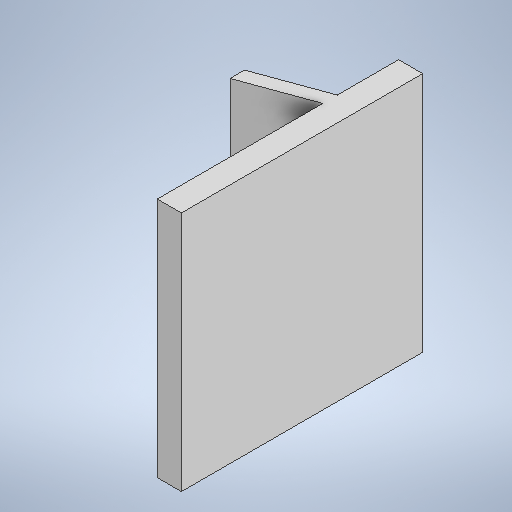
# Autodesk Inventor part: horony_upper
Saved by Autodesk Inventor 2025.2 (Build 292293000, 293)
## iProperties
Created: 2025-08-23
Part Number: horony_upper
Material: Generic
Document SubType Name: Modeling
Designer: MB
Density: 1 g/cm^3
Appearance: Default
Author: MB
Autodesk Inventor part; units mm, degrees
ref_plane "YZ Plane" through (0, 0, 0) normal (1, 0, 0) x (0, 1, 0)
ref_plane "XZ Plane" through (0, 0, 0) normal (0, 1, 0) x (-1, 0, 0)
ref_plane "XY Plane" through (0, 0, 0) normal (0, 0, 1) x (1, 0, 0)
sketch "Sketch4" plane through (0, 0, 0) normal (0, 1, 0) x (-1, 0, 0)
  line L0 (0, 0) -> (-5, 0)
  line L1 (-5, 0) -> (-5, -50)
  line L2 (-5, -50) -> (0, -50)
  line L3 (0, -50) -> (0, 0)
  line L4 (0, -37.3038) -> (14.0954, -32.1735)
  line L5 (0, -37.3038) -> (15, -37.3038) construction
  line L6 (14.0954, -32.1735) -> (14.0954, -29.1735)
  line L7 (14.0954, -29.1735) -> (0, -34.3038)
  dimension "d16" = 5
  dimension "d17" = 50
  dimension "d18" = 15
  dimension "d19" = 20
  dimension "d20" = 3
  constraints: 16 end point, 3 parallel, 2 horizontal, 2 point on line, 1 equal length, 1 perpendicular, 1 vertical
  measures "d16" distance of L2.end L1.end
  measures "d17" distance of L1.end L0.end
  measures "d18" distance of L4.start L4.end
  measures "d19" angle of L5 L4
  measures "d20" distance of L4.end L6.end
extrude "Extrusion3" add sketch "Sketch4" along normal blind 50
body "Solid2"
